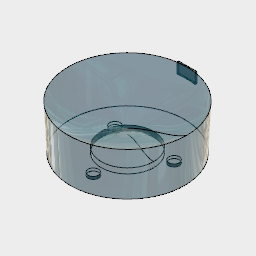
Side emitting lens v1 (Autodesk Fusion 360 design; units mm, degrees)
Autodesk Fusion 360 part; units mm, degrees
sketch "Sketch2" plane through (0, 0, 0) normal (0, 1, 0) x (1, 0, 0)
  line L0 (5, 0) -> (10.9, 0)
  line L1 (10.9, 0) -> (11.3, -8.5)
  line L2 (5, 0) -> (5, -1)
  spline S0 degree 5 poles (0, -3) (0.1093, -3) (0.3255, -2.9898) (0.6427, -2.9438) (1.0521, -2.8244) (1.5455, -2.5961) (2.026, -2.3122) (2.5, -2) (2.974, -1.6878) (3.4545, -1.4039) (3.9479, -1.1756) (4.3573, -1.0562) (4.6745, -1.0102) (4.8907, -1) (5, -1) knots 0 0 0 0 0 0 0.1 0.2 0.3 0.4 0.5 0.6 0.7 0.8 0.9 1 1 1 1 1 1
  line L3 (-0.5, -3) -> (0.5, -3)
  line L4 (4.5, -1) -> (5.5, -1)
  line L5 (0, -4) -> (0, -3)
  spline S1 degree 5 poles (11.3, -8.5) (11.0966, -8.3649) (10.6784, -8.1051) (10.0171, -7.7462) (9.0733, -7.3253) (7.8236, -6.8745) (6.5466, -6.4725) (5.2853, -6.0927) (4.0759, -5.7126) (2.9377, -5.3182) (1.8767, -4.9032) (1.0893, -4.5531) (0.5319, -4.2804) (0.1749, -4.0942) (0, -4) knots 0 0 0 0 0 0 0.1 0.2 0.3 0.4 0.5 0.6 0.7 0.8 0.9 1 1 1 1 1 1
  line L6 (12.422, -9.2449) -> (10.178, -7.7551)
  point P0 (2.5, -2)
  point P1 (5, -6)
  dimension "d2" = 10.9
  dimension "d5" = 11.3
  dimension "d7" = 1
  dimension "d14" = 3
  dimension "d15" = 4
  measures "d2" distance of origin L0.end
  measures "d5" distance of origin L1.end
  measures "d7" distance of L0.start L2.end
  measures "d14" distance of origin S0.start
  measures "d15" distance of origin L5.start
revolve "Revolve1" add sketch "Sketch2" angle 360 about axis through (0, 0, 1.75) along (0, 0, 1)
sketch "Sketch3" plane through (0, 0, 0) normal (0, 0, -1) x (1, 0, 0)
  circle A0 centre (0, 0) radius 5
  circle A1 centre (0, 0) radius 10.9
  circle A2 centre (0, 6.5) radius 1
  circle A3 centre (-5.6292, -3.25) radius 1
  circle A4 centre (5.6292, -3.25) radius 1
  dimension "d9" = 2
  dimension "d11" = 360
  measures "d9" diameter of A2
extrude "Extrude1" add sketch "Sketch3" along normal blind 0.5 contours A2 | A3 | A4
sketch "Sketch4" plane through (0, 0, 0) normal (0, 0, 1) x (1, 0, 0)
  line L0 (-1.75, 11.1) -> (1.75, 11.1)
  line L1 (1.75, 11.1) -> (1.75, 11.5)
  line L2 (1.75, 11.5) -> (-1.75, 11.5)
  line L3 (-1.75, 11.5) -> (-1.75, 11.1)
  circle A0 centre (0, 0) radius 11.3
  dimension "d16" = 3.5
  dimension "d17" = 1.75
  dimension "d18" = 11.5
  measures "d16" distance of L1.end L2.end
  measures "d17" distance of A0.centre L3
  measures "d18" distance of L2 A0.centre
extrude "Extrude2" add sketch "Sketch4" along normal blind 2 from surface at 6.5 contours L1 L2 L3 A0
equation "d2 = ( 21.8 / 2 ) * 1 mm"
equation "d5 = ( 22.6 / 2 ) * 1 mm"
equation "d17 = ( 3.5 / 2 ) * 1 mm"
equation "d18 = ( 23 / 2 ) * 1 mm"
